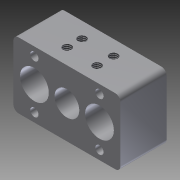
# Autodesk Inventor part: Mock Gearbox
Saved by Autodesk Inventor 2012 (Build 160160000, 160)
## iProperties
Created: 2013-01-19
Part Number: Mock Gearbox
Material: Default
Document SubType Name: Modeling
Designer: William
Density: 1 g/cm^3
Mass: 50.8415 g
Surface Area: 164.746 cm^2
Volume: 50.8415 cm^3
Author: William
Autodesk Inventor part; units mm, degrees
ref_plane "YZ Plane" through (0, 0, 0) normal (1, 0, 0) x (0, 1, 0)
ref_plane "XZ Plane" through (0, 0, 0) normal (0, 1, 0) x (-1, 0, 0)
ref_plane "XY Plane" through (0, 0, 0) normal (0, 0, 1) x (1, 0, 0)
sketch "Sketch1" plane through (0, 0, 0) normal (0, 0, 1) x (1, 0, 0)
  line L0 (-8.5249, 15.1341) -> (56.4751, 15.1341)
  line L1 (56.4751, 15.1341) -> (56.4751, -24.8659)
  line L2 (56.4751, -24.8659) -> (-8.5249, -24.8659)
  line L3 (-8.5249, -24.8659) -> (-8.5249, 15.1341)
  circle A0 centre (4.2251, -4.8659) radius 8.75
  line L4 (23.9751, 31.9095) -> (23.9751, -63.7078)
  circle A1 centre (43.7251, -4.8659) radius 8.75
  circle A2 centre (4.2251, 9.9285) radius 2.5
  circle A3 centre (4.2251, -19.471) radius 2.5
  circle A4 centre (43.7251, 9.9285) radius 2.5
  circle A5 centre (43.7251, -19.471) radius 2.5
  circle A6 centre (23.9751, -4.8659) radius 7.5
  point P0 (0, 0)
  dimension "d0" = 65
  dimension "d1" = 40
  dimension "d4" = 17.5
  dimension "d5" = 5
  dimension "d6" = 5
  dimension "d7" = 12.75
  dimension "d8" = 12.75
  dimension "d9" = 32.5
  dimension "d10" = 12.75
  dimension "d11" = 15
  constraints: 10 end point, 7 centre point, 3 parallel, 3 symmetric about line, 1 horizontal, 1 perpendicular, 1 point on line, 3 other
  measures "d0" distance of L0.start L0.end
  measures "d1" distance of L2.end L0.start
  measures "d4" diameter of A0
  measures "d5" diameter of A2
  measures "d6" diameter of A3
  measures "d7" distance from line of L3 A3.centre
  measures "d8" distance from line of L3 A0.centre
  measures "d9" distance between parallel lines of L4 L3
  measures "d10" distance from line of L3 A2.centre
  measures "d11" diameter of A6
extrude "Extrusion1" add sketch "Sketch1" along normal blind 28 contours L0 L4 A6 L2 L3 | L0 L1 L2 L4 A6
fillet "Fillet1" radius 3.175 4 edges at (-8.5249, 15.1341, 14) (56.4751, 15.1341, 14) (56.4751, -24.8659, 14) (-8.5249, -24.8659, 14)
sketch "Sketch2" plane through (-5.3499, 15.1341, 0) normal (0, 1, 0) x (1, 0, 0)
  line L0 (58.65, 0) -> (58.65, -28) projected
  line L1 (0, 0) -> (58.65, 0) projected
  line L2 (0, -28) -> (0, 0) projected
  line L3 (0, -28) -> (58.65, -28) projected
  circle A0 centre (20, -9.5) radius 2.5
  circle A1 centre (38.65, -9) radius 2.5
  line L4 (-22.4443, -14) -> (82.6683, -14)
  circle A2 centre (20, -18.5) radius 2.5
  circle A3 centre (38.65, -19) radius 2.5
  point P0 (5.3499, 0)
  dimension "d15" = 5
  dimension "d16" = 5
  dimension "d19" = 20
  dimension "d21" = 20
  dimension "d22" = 4.5
  dimension "d23" = 5
  dimension "d24" = 14
  dimension "d25" = 28
  constraints: 4 centre point, 2 end point, 2 symmetric about line, 1 parallel, 2 other
  measures "d15" diameter of A0
  measures "d16" diameter of A1
  measures "d19" distance from line of L2 A0.centre
  measures "d21" distance from line of L0 A1.centre
  measures "d22" distance from line of L4 A0.centre
  measures "d23" distance from line of L4 A1.centre
  measures "d24" distance between parallel lines of L1 L4
  measures "d25" distance of L2.start L1.start
extrude "Extrusion2" cut sketch "Sketch2" against normal blind 14 contours A0 | A1 | A2 | A3
thread "Thread1" size "12-24 UNC" class "2B" standard "ANSI Unified Screw Threads" full length
thread "Thread2" size "12-24 UNC" class "2B" standard "ANSI Unified Screw Threads" full length
thread "Thread3" size "12-24 UNC" class "2B" standard "ANSI Unified Screw Threads" full length
thread "Thread4" size "12-24 UNC" class "2B" standard "ANSI Unified Screw Threads" full length
equation "\"d7\" = d8"
equation "\"d10\" = d8"
equation "\"d21\" = d19"
equation "\"d23\" = d15"
equation "\"d24\" = 0.5 * d25"
body "Solid1"
